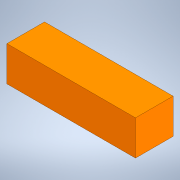
# Autodesk Inventor part: akksi
Saved by Autodesk Inventor 2020.2 (Build 242310000, 310)
## iProperties
Created: 2020-03-27
Part Number: akksi
Material: Generic
Document SubType Name: Modeling
Designer: Tarsoly
Density: 1 g/cm^3
Appearance: Default
Author: Tarsoly
Autodesk Inventor part; units mm, degrees
ref_plane "YZ Plane" through (0, 0, 0) normal (1, 0, 0) x (0, 1, 0)
ref_plane "XZ Plane" through (0, 0, 0) normal (0, 1, 0) x (-1, 0, 0)
ref_plane "XY Plane" through (0, 0, 0) normal (0, 0, 1) x (1, 0, 0)
sketch "Sketch1" plane through (0, 0, 0) normal (0, 1, 0) x (-1, 0, 0)
  line L0 (59, 17.25) -> (-59, 17.25)
  line L1 (-59, 17.25) -> (-59, -17.25)
  line L2 (-59, -17.25) -> (59, -17.25)
  line L3 (59, -17.25) -> (59, 17.25)
  line L4 (59, 17.25) -> (-59, -17.25) construction
  line L5 (-59, 17.25) -> (59, -17.25) construction
  point P0 (0, 0)
  dimension "d0" = 118
  dimension "d1" = 34.5
  constraints: 12 end point, 2 midpoint, 2 parallel, 1 horizontal, 1 perpendicular
  measures "d0" distance of L2.end L1.end
  measures "d1" distance of L1.end L0.end
extrude "Extrusion1" add sketch "Sketch1" along normal blind 32
body "Solid1"
